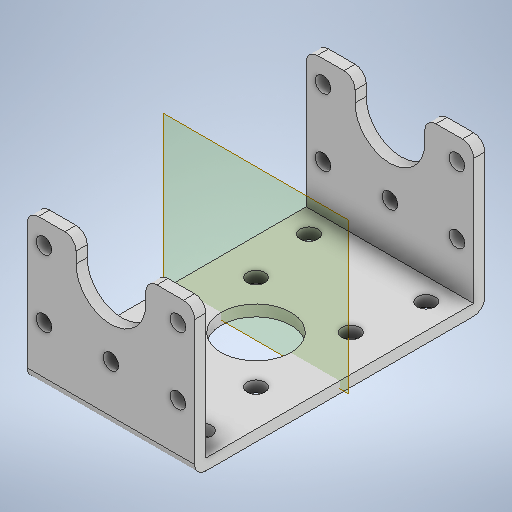
# Autodesk Inventor part: SmallerBracket
Saved by Autodesk Inventor 2027 (Build 310192060, 192F)
## iProperties
Created: 2026-07-11
Part Number: SmallerBracket
Material: Generic
Document SubType Name: Modeling
Designer: 13129
Density: 1 g/cm^3
Appearance: Default
Author: 13129
Autodesk Inventor part; units mm, degrees
ref_plane "YZ Plane" through (0, 0, 0) normal (1, 0, 0) x (0, 1, 0)
ref_plane "XZ Plane" through (0, 0, 0) normal (0, 1, 0) x (-1, 0, 0)
ref_plane "XY Plane" through (0, 0, 0) normal (0, 0, 1) x (1, 0, 0)
sketch "Sketch1" plane through (0, 0, 0) normal (0, 1, 0) x (-1, 0, 0)
  line L0 (0, 0) -> (-30, 0)
  line L1 (-30, 0) -> (-30, -48)
  line L2 (-30, -48) -> (0, -48)
  line L3 (0, -48) -> (0, 0)
  circle A0 centre (-15, -24) radius 6.25
  circle A1 centre (-23.5, -32.5) radius 1.6
  circle A2 centre (-6.5, -32.5) radius 1.6
  circle A3 centre (-4.5, -44) radius 1.6
  circle A4 centre (-25.5, -44) radius 1.6
  circle A5 centre (-23.5, -15.5) radius 1.6
  circle A6 centre (-6.5, -15.5) radius 1.6
  circle A7 centre (-4.5, -4) radius 1.6
  circle A8 centre (-25.5, -4) radius 1.6
  line L4 (-4.5, -44) -> (-25.5, -44) construction
  line L5 (-25.5, -44) -> (-25.5, -4) construction
  line L6 (-6.5, -32.5) -> (-23.5, -32.5) construction
  line L7 (-23.5, -32.5) -> (-23.5, -15.5) construction
  point P0 (0, -24)
  point P1 (-15, -48)
  point P2 (-23.5, -24)
  point P3 (-30, -24)
  point P4 (-25.5, -24)
  point P5 (-15, -32.5)
  point P6 (-15, -44)
  dimension "d0" = 30
  dimension "d1" = 48
  dimension "d2" = 12.5
  dimension "d3" = 3.2
  dimension "d4" = 17
  dimension "d5" = 17
  dimension "d6" = 40
  dimension "d7" = 21
  constraints: 16 end point, 9 centre point, 7 equal radius, 7 horizontal alignment, 7 midpoint, 7 vertical alignment, 4 perpendicular, 3 parallel, 1 horizontal
  measures "d0" distance of L2.end L1.end
  measures "d1" distance of L1.end L0.end
  measures "d2" diameter of A0
  measures "d3" diameter of A1
  measures "d4" distance of L6.start L6.end
  measures "d5" distance of L6.end L7.end
  measures "d6" distance of L4.end L5.end
  measures "d7" distance of L4.start L4.end
extrude "Extrusion1" add sketch "Sketch1" along normal blind 2
sketch "Sketch2" plane through (0, 0, 0) normal (0, 0, 1) x (1, 0, 0)
  line L0 (0, 0) -> (30, 0) construction
  line L1 (0, 0) -> (0, 24.5)
  line L2 (30, 0) -> (30, 24.5)
  arc A0 (8.75, 22.5) -> (21.25, 22.5) centre (15, 22.5) ccw
  line L3 (21.25, 22.5) -> (21.25, 24.5)
  line L4 (23.25, 26.5) -> (28, 26.5)
  line L5 (8.75, 22.5) -> (8.75, 24.5)
  line L6 (6.75, 26.5) -> (2, 26.5)
  arc A1 (8.75, 24.5) -> (6.75, 26.5) centre (6.75, 24.5) ccw
  arc A2 (2, 26.5) -> (0, 24.5) centre (2, 24.5) ccw
  arc A3 (30, 24.5) -> (28, 26.5) centre (28, 24.5) ccw
  arc A4 (23.25, 26.5) -> (21.25, 24.5) centre (23.25, 24.5) ccw
  circle A5 centre (27, 22.5) radius 1.4
  circle A6 centre (27, 10.5) radius 1.4
  circle A7 centre (15, 10.5) radius 1.4
  circle A8 centre (3, 10.5) radius 1.4
  circle A9 centre (3, 22.5) radius 1.4
  line L7 (3, 10.5) -> (27, 10.5) construction
  line L8 (0, 0) -> (30, 0)
  point P0 (0, 26.5)
  point P1 (30, 26.5)
  point P2 (15, 0)
  point P3 (15, 0)
  point P4 (15, 0)
  dimension "d10" = 26.5
  dimension "d11" = 26.5
  dimension "d12" = 12.5
  dimension "d13" = 22.5
  dimension "d14" = 2
  dimension "d15" = 2.8
  dimension "d16" = 12
  dimension "d17" = 24
  constraints: 16 end point, 10 centre point, 10 point on circle, 9 tangent, 7 equal radius, 5 vertical alignment, 4 horizontal alignment, 4 midpoint, 4 point on line, 4 vertical, 2 horizontal, 1 collinear, 1 parallel, 1 perpendicular
  measures "d10" distance of L0.start point (0, 26.5)
  measures "d11" distance of L0.end point (30, 26.5)
  measures "d12" diameter of A0
  measures "d13" vertical distance of L0.end A0.centre
  measures "d14" radius of A1
  measures "d15" diameter of A5
  measures "d16" distance of L7.start A9.centre
  measures "d17" distance of L7.start L7.end
extrude "Extrusion2" add sketch "Sketch2" along normal blind 2
fillet "Fillet1" radius 2 1 edges at (15, 0, 2)
ref_plane "Work Plane1" through (0, 0, -24) normal (0, 0, -1) x (-1, 0, 0)
sketch "Sketch3" plane through (0, 0, -24) normal (0, 0, -1) x (-1, 0, 0)
  point P0 (0, 0)
mirror "Mirror1" about plane through (0, 0, -24) normal (0, 0, -1) of "Extrusion2", "Fillet1"
body "Solid1"
